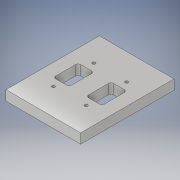
# Autodesk Inventor part: TFPX Plate
Saved by Autodesk Inventor 2019.4 (Build 234330000, 330)
## iProperties
Created: 2020-11-12
Part Number: TFPX Plate
Material: Generic
Document SubType Name: Modeling
Designer: caleb
Density: 1 g/cm^3
Appearance: Default
Author: caleb
Autodesk Inventor part; units mm, degrees
ref_plane "YZ Plane" through (0, 0, 0) normal (1, 0, 0) x (0, 1, 0)
ref_plane "XZ Plane" through (0, 0, 0) normal (0, 1, 0) x (-1, 0, 0)
ref_plane "XY Plane" through (0, 0, 0) normal (0, 0, 1) x (1, 0, 0)
sketch "Sketch1" plane through (0, 0, 0) normal (0, 1, 0) x (-1, 0, 0)
  line L0 (60, 75) -> (-60, 75)
  line L1 (-60, 75) -> (-60, -75)
  line L2 (-60, -75) -> (60, -75)
  line L3 (60, -75) -> (60, 75)
  point P0 (0, 0)
  dimension "d0" = 150
  dimension "d1" = 120
  dimension "d4" = 75
  dimension "d5" = 60
  constraints: 8 end point, 2 parallel, 1 horizontal, 1 perpendicular
  measures "d0" distance of L0.end L1.end
  measures "d1" distance of L0.start L0.end
  measures "d4" distance from line of L2 point (0, 0)
  measures "d5" distance from line of L1 point (0, 0)
extrude "Extrusion1" add sketch "Sketch1" along normal blind 15.875
sketch "Sketch2" plane through (0, 15.875, 0) normal (0, 1, 0) x (1, 0, 0)
  line L0 (-60, 75) -> (-60, -75) projected
  line L1 (-60, -75) -> (60, -75) projected
  circle A0 centre (-26.35, -32.5) radius 2.3813
  circle A1 centre (-26.35, 32.5) radius 2.3813
  circle A2 centre (26.35, -32.5) radius 2.3813
  circle A3 centre (26.35, 32.5) radius 2.3813
  point P0 (0, 0)
  dimension "d6" = 4.7625
  dimension "d7" = 33.65
  dimension "d8" = 4.7625
  dimension "d9" = 65
  dimension "d10" = 42.5
  constraints: 4 centre point, 1 vertical alignment
  measures "d6" diameter of A0
  measures "d7" distance from line of L0 A0.centre
  measures "d8" diameter of A1
  measures "d9" distance of A0.centre A1.centre
  measures "d10" distance from line of L1 A0.centre
hole "Hole1" at (-26.35, 15.875, -32.5) at (-26.35, 15.875, 32.5) at (26.35, 15.875, 32.5) at (26.35, 15.875, -32.5) direction (0, -1, 0) diameter 4.7625 depth 12.7 tip angle 118
sketch "Sketch3" plane through (0, 15.875, 0) normal (0, 1, 0) x (1, 0, 0)
  line L0 (-17.65, 20) -> (-35.05, 20)
  line L1 (-39.05, 16) -> (-39.05, -16)
  line L2 (-35.05, -20) -> (-17.65, -20)
  line L3 (-13.65, -16) -> (-13.65, 16)
  circle A0 centre (-26.35, 32.5) radius 2.3813 projected
  circle A1 centre (-26.35, -32.5) radius 2.3813 projected
  circle A2 centre (26.35, 32.5) radius 2.3813 projected
  circle A3 centre (26.35, -32.5) radius 2.3813 projected
  arc A4 (-13.65, 16) -> (-17.65, 20) centre (-17.65, 16) ccw
  arc A5 (-17.65, -20) -> (-13.65, -16) centre (-17.65, -16) ccw
  arc A6 (-39.05, -16) -> (-35.05, -20) centre (-35.05, -16) ccw
  arc A7 (-35.05, 20) -> (-39.05, 16) centre (-35.05, 16) ccw
  line L4 (17.65, 20) -> (35.05, 20)
  line L5 (39.05, 16) -> (39.05, -16)
  line L6 (35.05, -20) -> (17.65, -20)
  line L7 (13.65, -16) -> (13.65, 16)
  arc A8 (17.65, 20) -> (13.65, 16) centre (17.65, 16) ccw
  arc A9 (13.65, -16) -> (17.65, -20) centre (17.65, -16) ccw
  arc A10 (35.05, -20) -> (39.05, -16) centre (35.05, -16) ccw
  arc A11 (39.05, 16) -> (35.05, 20) centre (35.05, 16) ccw
  point P0 (0, 0)
  point P1 (-13.65, 20)
  point P2 (-39.05, 20)
  point P3 (-13.65, -20)
  point P4 (13.65, 20)
  point P5 (39.05, 20)
  point P6 (13.65, -20)
  point P7 (26.35, 32.5)
  point P8 (26.35, 32.5)
  dimension "d19" = 25.4
  dimension "d20" = 40
  dimension "d21" = 12.7
  dimension "d22" = 12.5
  dimension "d23" = 4
  constraints: 16 end point, 16 point on circle, 12 point on line, 8 centre point, 8 tangent, 3 equal radius, 2 parallel, 1 horizontal, 1 perpendicular
  measures "d19" distance of point (-13.65, 20) point (-39.05, 20)
  measures "d20" distance of point (-13.65, -20) point (-13.65, 20)
  measures "d21" distance from line of L3 point (-26.35, 32.5)
  measures "d22" distance from line of L0 point (-26.35, 32.5)
  measures "d23" radius of A4
extrude "Extrusion2" cut sketch "Sketch3" against normal blind 20 contours A4 L3 A5 L2 A6 L1 A7 L0 | L4 A11 L5 A10 L6 A9 L7 A8
sketch "Sketch4" plane through (0, 0, 0) normal (0, -1, 0) x (1, 0, 0)
  line L0 (-50, -61) -> (-50, 61)
  line L1 (-46, 65) -> (46, 65)
  line L2 (50, 61) -> (50, -61)
  line L3 (46, -65) -> (-46, -65)
  line L4 (-44, 35.5) -> (-44, -35.5)
  line L5 (-42, -37.5) -> (-11, -37.5)
  line L6 (-9, -35.5) -> (-9, 35.5)
  line L7 (-11, 37.5) -> (-42, 37.5)
  line L8 (11, -37.5) -> (42, -37.5)
  line L9 (44, -35.5) -> (44, 35.5)
  line L10 (42, 37.5) -> (11, 37.5)
  line L11 (9, 35.5) -> (9, -35.5)
  arc A0 (-50, -61) -> (-46, -65) centre (-46, -61) ccw
  arc A1 (-46, 65) -> (-50, 61) centre (-46, 61) ccw
  arc A2 (50, 61) -> (46, 65) centre (46, 61) ccw
  arc A3 (46, -65) -> (50, -61) centre (46, -61) ccw
  arc A4 (-44, -35.5) -> (-42, -37.5) centre (-42, -35.5) ccw
  arc A5 (-42, 37.5) -> (-44, 35.5) centre (-42, 35.5) ccw
  arc A6 (-9, 35.5) -> (-11, 37.5) centre (-11, 35.5) ccw
  arc A7 (-11, -37.5) -> (-9, -35.5) centre (-11, -35.5) ccw
  arc A8 (42, -37.5) -> (44, -35.5) centre (42, -35.5) ccw
  arc A9 (44, 35.5) -> (42, 37.5) centre (42, 35.5) ccw
  arc A10 (9, -35.5) -> (11, -37.5) centre (11, -35.5) ccw
  arc A11 (11, 37.5) -> (9, 35.5) centre (11, 35.5) ccw
  point P0 (0, 0)
  point P1 (-50, -65)
  point P2 (-50, 65)
  point P3 (50, 65)
  point P4 (-44, -37.5)
  point P5 (-9, -37.5)
  point P6 (9, -37.5)
  point P7 (44, -37.5)
  point P8 (44, 37.5)
  point P9 (9, 37.5)
  point P10 (-60, -75)
  point P11 (-60, 75)
  point P12 (60, 75)
  point P13 (60, -75)
  dimension "d26" = 10
  dimension "d27" = 10
  dimension "d28" = 10
  dimension "d29" = 10
  dimension "d30" = 75
  dimension "d31" = 35
  dimension "d32" = 4
  dimension "d33" = 27.5
  dimension "d34" = 6
  dimension "d35" = 6
  dimension "d36" = 35
  dimension "d37" = 2
  dimension "d38" = 2
  dimension "d39" = 2
  dimension "d40" = 2
  dimension "d41" = 2
  constraints: 24 end point, 24 point on circle, 24 tangent, 22 point on line, 12 centre point, 8 perpendicular, 6 equal radius, 2 vertical
  measures "d26" horizontal distance of point (-60, -75) point (-50, -65)
  measures "d27" horizontal distance of point (-60, -75) point (-50, -65)
  measures "d28" horizontal distance of point (-60, 75) point (-50, 65)
  measures "d29" horizontal distance of point (60, 75) point (50, 65)
  measures "d30" distance of point (9, 37.5) point (9, -37.5)
  measures "d31" distance of point (9, -37.5) point (44, -37.5)
  measures "d32" radius of A0
  measures "d33" distance between parallel lines of L8 L3
  measures "d34" distance between parallel lines of L2 L9
  measures "d35" distance between parallel lines of L0 L4
  measures "d36" distance of point (-44, -37.5) point (-9, -37.5)
  measures "d37" radius of A4
  measures "d38" radius of A8
  measures "d39" radius of A9
  measures "d40" radius of A10
  measures "d41" radius of A11
extrude "Extrusion3" cut sketch "Sketch4" against normal blind 10
body "Solid1"
